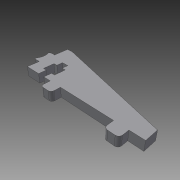
# Autodesk Inventor part: x_carryage_brace
Saved by Autodesk Inventor 2014 (Build 180170000, 170)
## iProperties
Created: 2014-02-23
Part Number: x_carryage_brace
Material: Generic
Document SubType Name: Modeling
Designer: buben
Density: 1 g/cm^3
Appearance: Default
Author: buben
Autodesk Inventor part; units mm, degrees
ref_plane "YZ Plane" through (0, 0, 0) normal (1, 0, 0) x (0, 1, 0)
ref_plane "XZ Plane" through (0, 0, 0) normal (0, 1, 0) x (-1, 0, 0)
ref_plane "XY Plane" through (0, 0, 0) normal (0, 0, 1) x (1, 0, 0)
sketch "Sketch1" plane through (0, 0, 0) normal (0, 0, 1) x (1, 0, 0)
  line L0 (0, 29) -> (0, 0)
  line L1 (0, 0) -> (78, 0)
  line L2 (78, 0) -> (78, 8)
  line L3 (78, 8) -> (4, 29)
  line L4 (4, 29) -> (0, 29)
  dimension "d0" = 29
  dimension "d1" = 78
  dimension "d2" = 4
  dimension "d3" = 8
  constraints: 10 end point, 2 parallel, 1 perpendicular, 1 vertical
  measures "d0" distance of L0.start L0.end
  measures "d1" distance of L0.end L1.end
  measures "d2" distance of L3.end L0.start
  measures "d3" distance of L1.end L2.end
extrude "Extrusion1" add sketch "Sketch1" along normal blind 6
sketch "Sketch2" plane through (0, 0, 6) normal (0, 0, 1) x (1, 0, 0)
  line L0 (0, 29) -> (0, 0) projected
  line L1 (0, 0) -> (78, 0) projected
  line L2 (78, 0) -> (78, 8) projected
  line L3 (4, 29) -> (0, 29) projected
  circle A0 centre (-11.099, 13.5) radius 7.5 construction
  line L4 (-6, 19) -> (-6, 8) construction
  arc A1 (-4.396, 9.5114) -> (-4.396, 17.4886) centre (-11.099, 13.5) ccw
  line L5 (-3.5366, 19) -> (0, 19)
  line L6 (-3.5366, 8) -> (0, 8)
  arc A2 (-3.5366, 19) -> (-4.396, 17.4886) centre (-3.5366, 18) ccw
  arc A3 (-4.396, 9.5114) -> (-3.5366, 8) centre (-3.5366, 9) ccw
  line L7 (20, 0) -> (28, 0)
  line L8 (28, 0) -> (28, -4)
  line L9 (26, -6) -> (22, -6)
  line L10 (20, -4) -> (20, 0)
  line L11 (62, 0) -> (70, 0)
  line L12 (70, 0) -> (70, -4)
  line L13 (68, -6) -> (64, -6)
  line L14 (62, -4) -> (62, 0)
  arc A4 (20, -4) -> (22, -6) centre (22, -4) ccw
  arc A5 (26, -6) -> (28, -4) centre (26, -4) ccw
  arc A6 (62, -4) -> (64, -6) centre (64, -4) ccw
  arc A7 (68, -6) -> (70, -4) centre (68, -4) ccw
  point P0 (-5.5682, 19)
  point P1 (-5.5682, 8)
  dimension "d6" = 15
  dimension "d7" = 11
  dimension "d8" = 6
  dimension "d9" = 11
  dimension "d10" = 7.8
  dimension "d11" = 10
  dimension "d12" = 1
  dimension "d13" = 2
  dimension "d15" = 8
  dimension "d17" = 8
  dimension "d18" = 6
  dimension "d19" = 20
  dimension "d20" = 8
  constraints: 22 end point, 18 point on circle, 12 tangent, 8 centre point, 6 point on line, 5 parallel, 5 perpendicular, 4 equal radius, 2 horizontal, 1 collinear
  measures "d6" diameter of A0
  measures "d7" distance of L4.start L4.end
  measures "d8" distance between parallel lines of L0 L4
  measures "d9" distance between parallel lines of L6 L5
  measures "d10" radius of A1
  measures "d11" distance between parallel lines of L3 L5
  measures "d12" radius of A2
  measures "d13" radius of A4
  measures "d15" distance between parallel lines of L8 L10
  measures "d17" distance between parallel lines of L12 L14
  measures "d18" distance between parallel lines of L1 L9
  measures "d19" distance between parallel lines of L0 L10
  measures "d20" distance between parallel lines of L2 L12
extrude "Extrusion2" add sketch "Sketch2" against normal blind 6
sketch "Sketch3" plane through (0, 0, 6) normal (0, 0, 1) x (1, 0, 0)
  line L0 (0, 0) -> (20, 0) projected
  line L1 (20, 0) -> (20, -4) projected
  line L2 (10.25, 16.3) -> (14.75, 16.3)
  line L3 (14.75, 0) -> (10.25, 0)
  line L4 (17.25, 12.3) -> (17.25, 5)
  line L5 (7.75, 5) -> (7.75, 12.3)
  line L6 (7.75, 12.3) -> (10.25, 12.3)
  line L7 (14.75, 12.3) -> (17.25, 12.3)
  line L8 (17.25, 5) -> (14.75, 5)
  line L9 (10.25, 5) -> (7.75, 5)
  line L10 (10.25, 0) -> (10.25, 5)
  line L11 (10.25, 12.3) -> (10.25, 16.3)
  line L12 (14.75, 16.3) -> (14.75, 12.3)
  line L13 (14.75, 5) -> (14.75, 0)
  point P0 (12.5, 16.3)
  dimension "d23" = 4.5
  dimension "d24" = 2.5
  dimension "d25" = 2.5
  dimension "d26" = 4
  dimension "d27" = 5
  dimension "d28" = 7.3
  dimension "d29" = 7.5
  constraints: 24 end point, 10 parallel, 5 collinear, 4 perpendicular, 3 horizontal, 1 midpoint
  measures "d23" distance of L2.start L2.end
  measures "d24" distance of L5.end L6.end
  measures "d25" distance of L7.start L4.start
  measures "d26" distance of L6.end L2.start
  measures "d27" distance of L3.end L9.start
  measures "d28" distance of L5.start L5.end
  measures "d29" distance from line of L1 point (12.5, 16.3)
extrude "Extrusion3" cut sketch "Sketch3" against normal through all
body "Solid1"
